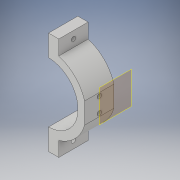
# Autodesk Inventor part: spannringe
Saved by Autodesk Inventor 2017 (Build 210142000, 142)
## iProperties
Part Number: spannringe
Material: Generisch
Document SubType Name: Modeling
Designer: Fabio
Density: 1 g/cm^3
Appearance: Vorgabe
Author: Fabio
Autodesk Inventor part; units mm, degrees
ref_plane "YZ Plane" through (0, 0, 0) normal (1, 0, 0) x (0, 1, 0)
ref_plane "XZ Plane" through (0, 0, 0) normal (0, 1, 0) x (-1, 0, 0)
ref_plane "XY Plane" through (0, 0, 0) normal (0, 0, 1) x (1, 0, 0)
sketch "Skizze1" plane through (0, 0, 0) normal (0, 1, 0) x (-1, 0, 0)
  arc A0 (-0.3929, 20.4962) -> (-20.5, 0) centre (0, 0) ccw
  arc A1 (-7.3929, 24.9268) -> (-26, 0) centre (0, 0) ccw
  line L0 (-0.3929, 20.4962) -> (-0.3929, 34.9962)
  line L1 (-0.3929, 34.9962) -> (-7.3929, 34.9962)
  line L2 (-7.3929, 34.9962) -> (-7.3929, 24.9268)
  line L3 (0, 0) -> (-16.7346, 0) construction
  arc A2 (-20.5, 0) -> (-0.3929, -20.4962) centre (0, 0) ccw
  arc A3 (-26, 0) -> (-7.3929, -24.9268) centre (0, 0) ccw
  line L4 (-0.3929, -20.4962) -> (-0.3929, -34.9962)
  line L5 (-0.3929, -34.9962) -> (-7.3929, -34.9962)
  line L6 (-7.3929, -34.9962) -> (-7.3929, -24.9268)
  dimension "d5" = 14.5
  dimension "d6" = 20.5
  dimension "d8" = 10.0694
  dimension "d9" = 7
  dimension "d51" = 26
  constraints: 14 end point, 8 point on circle, 4 centre point, 4 symmetric about line, 3 coincident, 2 perpendicular, 1 horizontal, 1 vertical, 2 other
  measures "d5" distance of L0.start L0.end
  measures "d6" radius of A0
  measures "d8" distance of L1.end L2.end
  measures "d9" distance of L0.end L1.end
  measures "d51" radius of A3
extrude "Extrusion1" add sketch "Skizze1" along normal blind 20
sketch "Skizze2" plane through (0.3929, 0, 20.4962) normal (-1, 0, 0) x (0, 0, 1)
  line L0 (14.5, 0) -> (14.5, 20) projected
  line L1 (14.5, 10) -> (-98.2028, 10) construction
  line L2 (0, 20) -> (14.5, 20) projected
  line L3 (-55.4925, 0) -> (-55.4925, 20) projected
  point P0 (-20.4962, 0)
  point P1 (9.5, 10)
  point P2 (-50.4925, 10)
  dimension "d12" = 10
  dimension "d13" = 5
  dimension "d14" = 5
  constraints: 2 end point, 2 point on line, 1 horizontal, 1 midpoint
  measures "d12" distance between parallel lines of L2 L1
  measures "d13" distance from line of point (9.5, 10) L0
  measures "d14" distance from line of L3 point (-50.492, 10)
hole "Bohrung1" at (0.3929, 10, 29.9962) at (0.3929, 10, -29.9962) direction (1, 0, 0) diameter 3 end through all
ref_plane "Arbeitsebene1" through (26, 20, 0) normal (1, 0, 0) x (0, 1, 0)
sketch "Skizze3" plane through (26, 20, 0) normal (1, 0, 0) x (0, 1, 0)
  line L0 (0, 20.4962) -> (0, -20.4962) projected
  line L1 (0, 15) -> (-20, 15)
  line L2 (-20, 15) -> (-20, -15)
  line L3 (-20, -15) -> (0, -15)
  line L4 (0, -15) -> (0, 15)
  point P0 (-20, 0)
  dimension "d28" = 20
  dimension "d30" = 15
  dimension "d31" = 15
  constraints: 8 end point, 2 parallel, 1 horizontal, 1 perpendicular, 1 point on line
  measures "d28" distance between parallel lines of L0 L2
  measures "d30" distance from line of L3 point (-20, 0)
  measures "d31" distance of L1.end point (-20, 0)
extrude "Extrusion2" cut sketch "Skizze3" against normal blind 1
sketch "Skizze4" plane through (26, 20, 0) normal (1, 0, 0) x (0, 1, 0)
  line L0 (0, -7.1414) -> (-20, -7.1414) construction
  line L1 (-10, -7.1414) -> (-10, 7.1414) construction
  line L2 (-20, 7.1414) -> (0, 7.1414) construction
  line L3 (-20, 0) -> (0, 0) construction
  line L4 (0, 20.4962) -> (0, -20.4962) construction
  point P0 (-10, -5)
  point P1 (-10, 5)
  dimension "d49" = 5
  dimension "d50" = 5
  constraints: 4 end point, 3 midpoint, 2 point on line
  measures "d49" distance from line of L3 point (-10, -5)
  measures "d50" distance from line of L3 point (-10, 5)
hole "Bohrung2" at (26, 10, -5) at (26, 10, 5) direction (-1, 0, 0) diameter 3 end through all
chamfer "Fase2" distance 1 angle 45 1 edges at (20.1824, 9.4756, -3.5947)
chamfer "Fase3" distance 1 angle 45 1 edges at (19.4422, 9.9997, 6.5)
